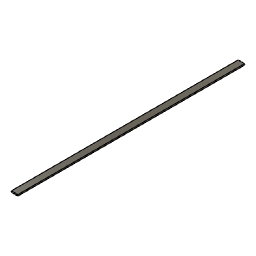
_Plaskownik20x4_700mm.b7b6e418-85cd-48e1-898f-45b313e5e4af (Autodesk Fusion 360 design; units mm, degrees)
Autodesk Fusion 360 part; units mm, degrees
sketch "Sketch1" plane through (0, 0, 0) normal (0, 1, 0) x (1, 0, 0)
  line L0 (0, -2) -> (10, -2)
  line L1 (10, -2) -> (10, 2)
  line L2 (10, 2) -> (0, 2)
  line L3 (0, -2) -> (-10, -2)
  line L4 (-10, -2) -> (-10, 2)
  line L5 (-10, 2) -> (0, 2)
  dimension "d1" = 10
  dimension "d2" = 4
  constraint horizontal L0
  constraint vertical L1
  constraint horizontal L2
  measures "d1" distance of L0.start L0.end
  measures "d2" distance of L0.start L2.end
extrude "Extrude1" add sketch "Sketch1" along normal blind 700
